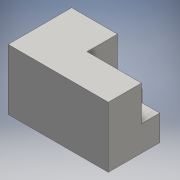
# Autodesk Inventor part: 240503_3Dsketch03
Saved by Autodesk Inventor 2016 (Build 200138000, 138)
## iProperties
Created: 2024-05-03
Part Number: 240503_3Dsketch03
Material: 일반
Document SubType Name: Modeling
Designer: pc
Density: 1 g/cm^3
Appearance: 기본값
Author: pc
Autodesk Inventor part; units mm, degrees
ref_plane "YZ Plane" through (0, 0, 0) normal (1, 0, 0) x (0, 1, 0)
ref_plane "XZ Plane" through (0, 0, 0) normal (0, 1, 0) x (-1, 0, 0)
ref_plane "XY Plane" through (0, 0, 0) normal (0, 0, 1) x (1, 0, 0)
sketch "스케치1" plane through (0, 0, 0) normal (0, 0, 1) x (1, 0, 0)
  line L0 (82.4719, -52.3014) -> (-82.4719, -52.3014)
  line L1 (-82.4719, -52.3014) -> (-82.4719, 52.3014)
  line L2 (-82.4719, 52.3014) -> (82.4719, 52.3014)
  line L3 (82.4719, 52.3014) -> (82.4719, -52.3014)
  line L4 (82.4719, -52.3014) -> (-82.4719, 52.3014) construction
  line L5 (-82.4719, -52.3014) -> (82.4719, 52.3014) construction
  point P0 (0, 0)
  constraints: 12 end point, 2 midpoint, 2 parallel, 1 horizontal, 1 perpendicular
extrude "돌출1" add sketch "스케치1" along normal blind 100
sketch "스케치2" plane through (-82.4719, 52.3014, 0) normal (0, 1, 0) x (1, 0, 0)
  line L0 (164.9439, 0) -> (0, 0) projected
  line L1 (164.9439, 0) -> (116.2257, 0)
  line L2 (116.2257, 0) -> (116.2257, -42.2338)
  line L3 (116.2257, -42.2338) -> (164.9439, -42.2338)
  line L4 (164.9439, -42.2338) -> (164.9439, 0)
  point P0 (82.4719, 0)
  constraints: 8 end point, 2 parallel, 1 horizontal, 1 perpendicular
extrude "돌출2" cut sketch "스케치2" against normal blind 20
sketch "스케치3" plane through (-82.4719, 52.3014, 100) normal (0, 1, 0) x (1, 0, 0)
  line L0 (164.9439, 0) -> (0, 0) projected
  line L1 (164.9439, 57.7662) -> (116.2257, 57.7662) projected
  line L2 (75.3221, 0) -> (164.9439, 0)
  line L3 (164.9439, 0) -> (164.9439, 57.7662)
  line L4 (164.9439, 57.7662) -> (75.3221, 57.7662)
  line L5 (75.3221, 57.7662) -> (75.3221, 0)
  point P0 (82.4719, 100)
  constraints: 8 end point, 2 parallel, 1 horizontal, 1 perpendicular, 1 point on line
extrude "돌출3" cut sketch "스케치3" against normal blind 50
